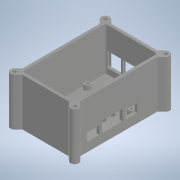
# Autodesk Inventor part: Test
Saved by Autodesk Inventor 2021 (Build 250183000, 183)
## iProperties
Created: 2021-07-24
Part Number: Test
Material: ABS Plastic
Document SubType Name: Modeling
Designer: cmzgt
Density: 0.1 g/cm^3
Appearance: Smooth - White
Author: cmzgt
Autodesk Inventor part; units mm, degrees
ref_plane "YZ Plane" through (0, 0, 0) normal (1, 0, 0) x (0, 1, 0)
ref_plane "XZ Plane" through (0, 0, 0) normal (0, 1, 0) x (-1, 0, 0)
ref_plane "XY Plane" through (0, 0, 0) normal (0, 0, 1) x (1, 0, 0)
sketch "Sketch1" plane through (0, 0, 0) normal (0, 1, 0) x (-1, 0, 0)
  line L0 (-31.93, -49.55) -> (31.93, -49.55)
  line L1 (31.93, -49.55) -> (31.93, 49.55)
  line L2 (31.93, 49.55) -> (-31.93, 49.55)
  line L3 (-31.93, 49.55) -> (-31.93, -49.55)
  line L4 (-31.93, -49.55) -> (31.93, 49.55) construction
  line L5 (31.93, -49.55) -> (-31.93, 49.55) construction
  point P0 (0, 0)
  dimension "d0" = 63.86
  dimension "d1" = 99.1
  constraints: 12 end point, 2 midpoint, 2 parallel, 1 horizontal, 1 perpendicular
  measures "d0" distance of L2.end L1.end
  measures "d1" distance of L0.end L1.end
extrude "Extrusion1" add sketch "Sketch1" along normal blind 5.08
sketch "Sketch2" plane through (0, 5.08, 0) normal (0, 1, 0) x (1, 0, 0)
  line L0 (28.73, 46.35) -> (-28.73, 46.35)
  line L1 (-28.73, 46.35) -> (-28.73, -46.35)
  line L2 (-28.73, -46.35) -> (28.73, -46.35)
  line L3 (28.73, -46.35) -> (28.73, 46.35)
  line L4 (28.73, 46.35) -> (-28.73, -46.35) construction
  line L5 (-28.73, 46.35) -> (28.73, -46.35) construction
  line L6 (-31.93, 49.55) -> (-31.93, -49.55) projected
  line L7 (-31.93, -49.55) -> (31.93, -49.55) projected
  line L8 (31.93, 49.55) -> (-31.93, 49.55) projected
  line L9 (31.93, -49.55) -> (31.93, 49.55) projected
  line L10 (25.53, -43.15) -> (31.93, -49.55) construction
  line L11 (23.0731, -46.35) -> (29.1016, -52.3784)
  line L12 (34.7584, -46.7216) -> (28.73, -40.6931)
  arc A0 (29.1016, -52.3784) -> (34.7584, -46.7216) centre (31.93, -49.55) ccw
  circle A1 centre (31.93, -49.55) radius 1.375
  point P0 (0, 0)
  dimension "d4" = 3.2
  dimension "d5" = 3.2
  dimension "d22" = 8
  dimension "d23" = 2.75
  constraints: 20 end point, 4 parallel, 3 midpoint, 2 centre point, 2 point on circle, 2 point on line, 2 tangent, 1 coincident, 1 horizontal, 1 perpendicular
  measures "d4" distance between parallel lines of L6 L1
  measures "d5" distance between parallel lines of L7 L2
  measures "d22" diameter of A0
  measures "d23" diameter of A1
extrude "Extrusion2" add sketch "Sketch2" along normal blind 48 contours L0 L1 L2 L11 L7 L6 L8 L9 L12 L3 | L12 L9 A1 L7 L11 L2 L3 | L9 L7 A1 picked at (31.2859, -48.9059)
sketch "Sketch3" plane through (0, 5.08, 0) normal (0, 1, 0) x (1, 0, 0)
  line L0 (28.73, -46.35) -> (-28.73, -46.35) construction
  line L1 (0, -46.35) -> (0, 46.35) construction
  line L2 (28.73, 46.35) -> (-28.73, 46.35) construction
  circle A0 centre (-24.5, -36.35) radius 3.5
  circle A1 centre (-24.5, -36.35) radius 1.375
  line L3 (28.73, 46.35) -> (28.73, -46.35) construction
  line L4 (28.73, 0) -> (-28.73, 0) construction
  line L5 (-28.73, -46.35) -> (-28.73, 46.35) construction
  circle A2 centre (-24.5, 21.65) radius 3.5
  circle A3 centre (-24.5, 21.65) radius 1.375
  circle A4 centre (24.5, -36.35) radius 3.5
  circle A5 centre (24.5, -36.35) radius 1.375
  circle A6 centre (24.5, 21.65) radius 3.5
  circle A7 centre (24.5, 21.65) radius 1.375
  point P0 (0, 0)
  dimension "d8" = 7
  dimension "d9" = 2.75
  dimension "d10" = 10
  dimension "d11" = 24.5
  dimension "d14" = 58
  constraints: 8 centre point, 4 coincident, 4 end point, 4 midpoint, 4 symmetric about line, 1 vertical, 8 other
  measures "d8" diameter of A0
  measures "d9" diameter of A1
  measures "d10" distance from line of L0 A0.centre
  measures "d11" distance from line of L1 A1.centre
  measures "d14" distance of A0.centre A2.centre
extrude "Extrusion3" add sketch "Sketch3" along normal blind 5
sketch "Sketch4" plane through (0, 0, 0) normal (0, -1, 0) x (1, 0, 0)
  line L0 (29.6707, 47.5763) -> (34.1893, 51.5237) construction
  line L1 (31.93, 49.55) -> (31.93, -49.55) projected
  line L2 (31.93, 43.5747) -> (37.1499, 48.1348)
  line L3 (31.2287, 54.9127) -> (26.7101, 50.9652)
  arc A0 (26.7101, 50.9652) -> (25.6267, 49.55) centre (29.6707, 47.5763) ccw
  arc A1 (37.1499, 48.1348) -> (31.2287, 54.9127) centre (34.1893, 51.5237) ccw
  line L4 (-31.93, 49.55) -> (31.93, 49.55) projected
  line L5 (25.6267, 49.55) -> (31.93, 49.55)
  line L6 (31.93, 49.55) -> (31.93, 43.5747)
  circle A2 centre (34.1893, 51.5237) radius 1.85
  line L7 (0, 49.55) -> (0, -49.55) construction
  line L8 (31.93, -49.55) -> (-31.93, -49.55) construction
  line L9 (31.93, 0) -> (-33.3, 0) construction
  line L10 (31.93, -49.55) -> (31.93, 49.55)
  line L11 (31.93, -43.5747) -> (37.1499, -48.1348)
  line L12 (31.2287, -54.9127) -> (26.7101, -50.9652)
  arc A3 (25.6267, -49.55) -> (26.7101, -50.9652) centre (29.6707, -47.5763) ccw
  arc A4 (31.2287, -54.9127) -> (37.1499, -48.1348) centre (34.1893, -51.5237) ccw
  line L13 (-31.93, -49.55) -> (31.93, -49.55)
  circle A5 centre (34.1893, -51.5237) radius 1.85
  line L14 (-31.93, 49.55) -> (-31.93, -49.55)
  line L15 (-31.93, 43.5747) -> (-37.1499, 48.1348)
  line L16 (-31.2287, 54.9127) -> (-26.7101, 50.9652)
  arc A6 (-25.6267, 49.55) -> (-26.7101, 50.9652) centre (-29.6707, 47.5763) ccw
  arc A7 (-31.2287, 54.9127) -> (-37.1499, 48.1348) centre (-34.1893, 51.5237) ccw
  line L17 (-25.6267, 49.55) -> (-31.93, 49.55)
  circle A8 centre (-34.1893, 51.5237) radius 1.85
  arc A9 (-37.1499, -48.1348) -> (-31.2287, -54.9127) centre (-34.1893, -51.5237) ccw
  line L18 (-31.93, -43.5747) -> (-37.1499, -48.1348)
  line L19 (-31.2287, -54.9127) -> (-26.7101, -50.9652)
  arc A10 (-26.7101, -50.9652) -> (-25.6267, -49.55) centre (-29.6707, -47.5763) ccw
  circle A11 centre (-34.1893, -51.5237) radius 1.85
  line L20 (-25.6267, -49.55) -> (-31.93, -49.55)
  line L21 (-31.93, -49.55) -> (-31.93, 49.55)
  point P0 (0, 0)
  point P1 (-31.93, -43.5747)
  point P2 (31.93, -43.5747)
  point P3 (31.93, -49.55)
  dimension "d24" = 3
  dimension "d25" = 9
  dimension "d26" = 131.141
  dimension "d27" = 3.7
  constraints: 40 end point, 30 symmetric about line, 16 point on circle, 12 centre point, 6 point on line, 4 coincident, 4 midpoint, 4 tangent, 1 collinear, 1 horizontal, 1 parallel, 9 other
  measures "d24" distance of L1.start L0.end
  measures "d25" diameter of A1
  measures "d26" angle of L1 L2
  measures "d27" diameter of A2
extrude "Extrusion4" add sketch "Sketch4" against normal up to surface (53.08 mm away) contours L4 A0 L3 A1 L2 L1 | L11 A4 L12 A3 L13 L1 | L4 L14 L15 A7 L16 A6 | A10 L19 A9 L18 L14 L13
fillet "Fillet2" radius 2 4 edges at (28.73, 29.08, -46.35) (-28.73, 29.08, -46.35) (-28.73, 29.08, 46.35) (28.73, 29.08, 46.35)
sketch "Sketch5" plane through (0, 5.08, 0) normal (0, 1, 0) x (1, 0, 0)
  line L0 (15, 0) -> (-15, 0) construction
  line L1 (15, 2.5) -> (-15, 2.5)
  line L2 (-15, -2.5) -> (15, -2.5)
  arc A0 (15, -2.5) -> (15, 2.5) centre (15, 0) ccw
  arc A1 (-15, 2.5) -> (-15, -2.5) centre (-15, 0) ccw
  line L3 (-26.73, -46.35) -> (26.73, -46.35) construction
  line L4 (0, -46.35) -> (0, 46.35) construction
  line L5 (-26.73, 46.35) -> (26.73, 46.35) construction
  arc A2 (-15, 12.5) -> (-15, 7.5) centre (-15, 10) ccw
  line L6 (15, 12.5) -> (-15, 12.5)
  line L7 (-15, 7.5) -> (15, 7.5)
  arc A3 (15, 7.5) -> (15, 12.5) centre (15, 10) ccw
  arc A4 (-15, 22.5) -> (-15, 17.5) centre (-15, 20) ccw
  line L8 (15, 22.5) -> (-15, 22.5)
  line L9 (-15, 17.5) -> (15, 17.5)
  arc A5 (15, 17.5) -> (15, 22.5) centre (15, 20) ccw
  arc A6 (-15, 32.5) -> (-15, 27.5) centre (-15, 30) ccw
  line L10 (15, 32.5) -> (-15, 32.5)
  line L11 (-15, 27.5) -> (15, 27.5)
  arc A7 (15, 27.5) -> (15, 32.5) centre (15, 30) ccw
  arc A8 (-15, -7.5) -> (-15, -12.5) centre (-15, -10) ccw
  line L12 (-15, -12.5) -> (15, -12.5)
  line L13 (15, -7.5) -> (-15, -7.5)
  arc A9 (15, -12.5) -> (15, -7.5) centre (15, -10) ccw
  arc A10 (-15, -17.5) -> (-15, -22.5) centre (-15, -20) ccw
  line L14 (-15, -22.5) -> (15, -22.5)
  line L15 (15, -17.5) -> (-15, -17.5)
  arc A11 (15, -22.5) -> (15, -17.5) centre (15, -20) ccw
  arc A12 (-15, -27.5) -> (-15, -32.5) centre (-15, -30) ccw
  line L16 (-15, -32.5) -> (15, -32.5)
  line L17 (15, -27.5) -> (-15, -27.5)
  arc A13 (15, -32.5) -> (15, -27.5) centre (15, -30) ccw
  point P0 (0, 0)
  dimension "d31" = 15
  dimension "d32" = 5
  dimension "d35" = 10
  dimension "d42" = 10
  constraints: 34 end point, 28 point on circle, 14 centre point, 4 tangent, 3 midpoint, 2 vertical, 1 horizontal, 1 parallel, 60 other
  measures "d31" distance of point (0, 0) L0.end
  measures "d32" diameter of A1
  measures "d35" distance of L0.end A2.centre
  measures "d42" distance of L0.end A8.centre
extrude "Extrusion5" cut sketch "Sketch5" against normal up to surface (5.08 mm away)
sketch "Sketch12" plane through (31.93, 0, 43.5747) normal (1, 0, 0) x (0, 0, -1)
  line L0 (0, 53.08) -> (0, 0) projected
  line L1 (28.1666, 16.69) -> (28.1666, 14.2116) projected
  line L2 (43.1666, 14.2116) -> (43.1666, 16.69) projected
  line L3 (10.2763, 12.8971) -> (10.2763, 13.09) projected
  line L4 (18.257, 13.09) -> (18.257, 12.8971) projected
  line L5 (53.7666, 17.41) -> (53.7666, 11.41) projected
  line L6 (60.7666, 11.41) -> (60.7666, 17.41) projected
  line L7 (11.2666, 14.1354) -> (17.2666, 14.1354) projected
  line L8 (21.0747, 5.08) -> (26.0747, 5.08) projected
  line L9 (26.0747, 5.08) -> (21.0747, 5.08) projected
  line L10 (41.0747, 5.08) -> (46.0747, 5.08) projected
  line L11 (46.0747, 5.08) -> (41.0747, 5.08) projected
  line L12 (51.0747, 5.08) -> (56.0747, 5.08) projected
  line L13 (56.0747, 5.08) -> (51.0747, 5.08) projected
  line L14 (61.0747, 5.08) -> (66.0747, 5.08) projected
  line L15 (66.0747, 5.08) -> (61.0747, 5.08) projected
  line L16 (11.0747, 5.08) -> (16.0747, 5.08) projected
  line L17 (16.0747, 5.08) -> (11.0747, 5.08) projected
  line L18 (31.0747, 5.08) -> (36.0747, 5.08) projected
  line L19 (36.0747, 5.08) -> (31.0747, 5.08) projected
  line L20 (71.0747, 5.08) -> (76.0747, 5.08) projected
  line L21 (76.0747, 5.08) -> (71.0747, 5.08) projected
  line L22 (3.7247, 5.08) -> (10.7247, 5.08) projected
  line L23 (3.7247, 5.08) -> (10.7247, 5.08) projected
  line L24 (61.7247, 5.08) -> (68.7247, 5.08) projected
  line L25 (61.7247, 5.08) -> (68.7247, 5.08) projected
  line L26 (-2.7753, 5.08) -> (-0.7753, 5.08) projected
  line L27 (-0.7753, 5.08) -> (87.9247, 5.08) projected
  line L28 (87.9247, 5.08) -> (89.9247, 5.08) projected
  line L29 (89.9247, 5.08) -> (87.9247, 5.08) projected
  line L30 (87.9247, 5.08) -> (-0.7753, 5.08) projected
  line L31 (-0.7753, 5.08) -> (-2.7753, 5.08) projected
  line L32 (5.8497, 10.08) -> (8.5997, 10.08) projected
  line L33 (10.2763, 12.9936) -> (18.257, 12.9936) construction
  line L34 (14.2666, 14.1354) -> (14.2666, 12.9936) construction
  line L35 (7.2763, 19.08) -> (21.257, 19.08)
  line L36 (21.257, 19.08) -> (21.257, 10.08)
  line L37 (21.257, 10.08) -> (7.2763, 10.08)
  line L38 (7.2763, 10.08) -> (7.2763, 19.08)
  line L39 (42.3666, 17.49) -> (28.9666, 17.49) projected
  line L40 (47.1666, 10.08) -> (24.1666, 10.08)
  line L41 (24.1666, 10.08) -> (24.1666, 22.08)
  line L42 (24.1666, 22.08) -> (47.1666, 22.08)
  line L43 (47.1666, 22.08) -> (47.1666, 10.08)
  line L44 (60.7666, 17.41) -> (57.2666, 17.41) projected
  line L45 (63.7666, 10.08) -> (50.7666, 10.08)
  line L46 (50.7666, 10.08) -> (50.7666, 19.68)
  line L47 (50.7666, 19.68) -> (63.7666, 19.68)
  line L48 (63.7666, 19.68) -> (63.7666, 10.08)
  point P0 (43.5747, 0)
  dimension "d99" = 3
  dimension "d100" = 3
  dimension "d101" = 0
  dimension "d102" = 9
  dimension "d103" = 4
  dimension "d104" = 4
  dimension "d105" = 0
  dimension "d106" = 12
  dimension "d108" = 3
  dimension "d109" = 3
  dimension "d110" = 0
  dimension "d111" = 9.6
  constraints: 28 end point, 6 parallel, 4 midpoint, 3 horizontal, 3 perpendicular
  measures "d99" distance from line of L4.end L36
  measures "d100" distance between parallel lines of L38 L3
  measures "d101" distance between parallel lines of L32 L37
  measures "d102" distance of L37.end L35.start
  measures "d103" distance between parallel lines of L43 L2
  measures "d104" distance between parallel lines of L41 L1
  measures "d105" distance between parallel lines of L32 L40
  measures "d106" distance of L40.end L41.end
  measures "d108" distance between parallel lines of L48 L6
  measures "d109" distance between parallel lines of L5 L46
  measures "d110" distance between parallel lines of L32 L45
  measures "d111" distance of L45.end L46.end
extrude "Extrusion9" cut sketch "Sketch12" against normal up to surface (3.2 mm away)
sketch "Sketch14" plane through (25.6267, 0, -49.55) normal (0, 0, -1) x (-1, 0, 0)
  line L0 (0.5198, 11.61) -> (0.5198, 25.11) projected
  line L1 (16.3998, 11.61) -> (16.3998, 25.11) projected
  line L2 (0.5198, 25.11) -> (16.3998, 25.11) projected
  line L3 (0.5198, 11.61) -> (16.3998, 11.61) projected
  line L4 (0.5198, 18.36) -> (16.3998, 18.36) construction
  line L5 (16.8998, 11.11) -> (0.2698, 11.11)
  line L6 (0.2698, 11.11) -> (0.2698, 25.61)
  line L7 (0.2698, 25.61) -> (16.8998, 25.61)
  line L8 (16.8998, 25.61) -> (16.8998, 11.11)
  line L9 (24.2098, 27.1) -> (30.2098, 27.1) projected
  line L10 (34.7598, 21.3896) -> (34.7598, 18.3896) projected
  line L11 (19.6598, 18.3896) -> (19.6598, 21.3896) projected
  line L12 (25.6198, 11.41) -> (28.7998, 11.41) projected
  line L13 (35.2598, 10.91) -> (18.6659, 10.91)
  line L14 (18.6659, 10.91) -> (18.6659, 28.1)
  line L15 (18.6659, 28.1) -> (35.2598, 28.1)
  line L16 (35.2598, 28.1) -> (35.2598, 10.91)
  line L17 (19.1659, 18.3896) -> (19.1659, 21.3896) projected
  point P0 (25.6267, 0)
  dimension "d114" = 0.5
  dimension "d115" = 0.5
  dimension "d116" = 0.25
  dimension "d117" = 0.5
  dimension "d120" = 1
  dimension "d122" = 0.5
  dimension "d123" = 0.5
  dimension "d124" = 0.5
  constraints: 18 end point, 4 parallel, 2 horizontal, 2 midpoint, 2 perpendicular
  measures "d114" distance between parallel lines of L7 L2
  measures "d115" distance between parallel lines of L1 L8
  measures "d116" distance between parallel lines of L0 L6
  measures "d117" distance between parallel lines of L3 L5
  measures "d120" distance between parallel lines of L15 L9
  measures "d122" distance between parallel lines of L10 L16
  measures "d123" distance between parallel lines of L12 L13
  measures "d124" distance between parallel lines of L14 L17
extrude "Extrusion10" cut sketch "Sketch14" against normal up to surface (3.2 mm away) contours L0 L2 L1 L3 | L13 L14 L15 L16
body "Solid1"
